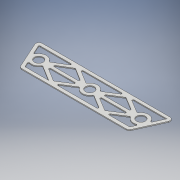
# Autodesk Inventor part: 6wdPlateInner
Saved by Autodesk Inventor 2018.3 (Build 223284000, 284)
## iProperties
Created: 2018-06-26
Part Number: 6wdPlateInner
Material: Generic
Document SubType Name: Modeling
Designer: mzhang
Density: 1 g/cm^3
Appearance: Default
Author: mzhang
Autodesk Inventor part; units mm, degrees
ref_plane "YZ Plane" through (0, 0, 0) normal (1, 0, 0) x (0, 1, 0)
ref_plane "XZ Plane" through (0, 0, 0) normal (0, 1, 0) x (-1, 0, 0)
ref_plane "XY Plane" through (0, 0, 0) normal (0, 0, 1) x (1, 0, 0)
sketch "Sketch1" plane through (0, 0, 0) normal (0, 0, 1) x (1, 0, 0)
  circle A0 centre (0, 0) radius 14.2875
  circle A1 centre (330.2, 0) radius 14.2875
  line L0 (-49.8896, 37.287) -> (-11.9465, -46.452)
  line L1 (-40.781, 51.4142) -> (51.1531, 51.4142) construction
  line L2 (-2.8379, -52.3248) -> (335.0491, -52.3248)
  line L3 (344.1679, -46.4293) -> (381.8605, 37.3096)
  line L4 (372.7417, 51.4142) -> (-40.781, 51.4142)
  circle A2 centre (165.1, 0) radius 14.2875
  arc A3 (-40.781, 51.4142) -> (-49.8896, 37.287) centre (-40.781, 41.4142) ccw
  arc A4 (-11.9465, -46.452) -> (-2.8379, -52.3248) centre (-2.8379, -42.3248) ccw
  arc A5 (335.0491, -52.3248) -> (344.1679, -46.4293) centre (335.0491, -42.3248) ccw
  arc A6 (381.8605, 37.3096) -> (372.7417, 51.4142) centre (372.7417, 41.4142) ccw
  line L5 (33.4321, 5) -> (131.8673, 5)
  line L6 (198.195, 5) -> (296.7702, 5)
  line L7 (33.2893, -5) -> (132.005, -5)
  line L8 (198.5298, -5) -> (297.105, -5)
  line L9 (330.2, 0) -> (315.9125, 0)
  arc A7 (-5.925, -23.5537) -> (20.7741, -12.5825) centre (0, 0) ccw
  arc A8 (20.7925, 12.5521) -> (-21.6765, 10.9549) centre (0, 0) ccw
  line L10 (0, 0) -> (14.2875, 0)
  arc A9 (142.9266, -9.9107) -> (187.2845, -9.886) centre (165.1, 0) ccw
  arc A10 (187.2734, 9.9107) -> (142.9218, 9.9) centre (165.1, 0) ccw
  arc A11 (354.4734, 0.8287) -> (308.0155, 9.886) centre (330.2, 0) ccw
  arc A12 (308.0266, -9.9107) -> (345.6741, -18.7199) centre (330.2, 0) ccw
  line L11 (372.7424, 41.7007) -> (354.4734, 0.8287)
  line L12 (345.6741, -18.7199) -> (335.1217, -41.2193)
  line L13 (-3.5725, -40.2425) -> (-9.3784, -27.7254)
  line L14 (-27.0783, 11.0519) -> (-38.8215, 36.5186)
  line L15 (24.9128, 11.5352) -> (64.4421, 35.4317)
  line L16 (92.8242, 41.0668) -> (142.9218, 9.9)
  line L17 (33.4321, 5) -> (83.3557, 35.1801)
  line L18 (83.3557, 35.1801) -> (131.8673, 5)
  line L19 (33.2893, -5) -> (83.3551, -35.8908)
  line L20 (83.3551, -35.8908) -> (132.005, -5)
  line L21 (24.9154, -11.5836) -> (73.9059, -41.8109)
  line L22 (92.7543, -41.7682) -> (142.9266, -9.9107)
  line L23 (187.2734, 9.9107) -> (236.8547, 41.393)
  line L24 (255.8424, 41.436) -> (308.0155, 9.886)
  line L25 (198.195, 5) -> (246.2801, 35.5322)
  line L26 (246.2801, 35.5322) -> (296.7702, 5)
  line L27 (198.5298, -5) -> (249.0199, -35.5322)
  line L28 (249.0199, -35.5322) -> (297.105, -5)
  line L29 (187.2845, -9.886) -> (239.4576, -41.436)
  line L30 (258.4453, -41.393) -> (308.0266, -9.9107)
  line L31 (-36.104, 40.7748) -> (62.8833, 40.999)
  line L32 (92.8242, 41.0668) -> (372.7424, 41.7007)
  line L33 (335.1217, -41.2193) -> (258.4453, -41.393)
  arc A13 (-27.0783, 11.0519) -> (-21.6765, 10.9549) centre (-24.354, 12.3081) ccw
  arc A14 (-36.104, 40.7748) -> (-38.8215, 36.5186) centre (-36.0972, 37.7748) ccw
  arc A15 (64.4421, 35.4317) -> (62.8833, 40.999) centre (62.8901, 37.999) ccw
  arc A16 (20.7925, 12.5521) -> (24.9128, 11.5352) centre (23.3608, 14.1025) ccw
  arc A17 (24.9154, -11.5836) -> (20.7741, -12.5825) centre (23.3401, -14.1367) ccw
  arc A18 (-5.925, -23.5537) -> (-9.3784, -27.7254) centre (-6.6569, -26.4631) ccw
  arc A19 (-3.5725, -40.2425) -> (-0.8442, -41.9802) centre (-0.851, -38.9802) ccw
  line L34 (239.4576, -41.436) -> (92.7543, -41.7682)
  line L35 (73.9059, -41.8109) -> (-0.8442, -41.9802)
  point P0 (-23.9208, 4.2044)
  point P1 (-12.6105, -20.7571)
  point P2 (22.1801, -9.8958)
  point P3 (22.1845, 9.8858)
  dimension "d0" = 28.575
  dimension "d9" = 10
  dimension "d22" = 3
  constraints: 72 end point, 38 point on circle, 23 tangent, 18 centre point, 13 parallel, 9 equal radius, 6 point on line, 2 horizontal, 2 horizontal alignment, 1 coincident, 1 equal length, 4 other
  measures "d9" radius of A3
  measures "d22" radius of A13
extrude "Extrusion1" add sketch "Sketch1" along normal blind 3.175
fillet "Fillet1" radius 3 26 edges at (33.4321, 5, 1.5875) (83.3557, 35.1801, 1.5875) (131.8673, 5, 1.5875) (33.2893, -5, 1.5875) (132.005, -5, 1.5875) (83.3551, -35.8908, 1.5875) (92.7543, -41.7682, 1.5875) (142.9266, -9.9107, 1.5875) (142.9218, 9.9, 1.5875) (92.8242, 41.0668, 1.5875) (236.8547, 41.393, 1.5875) (239.4576, -41.436, 1.5875) (187.2845, -9.886, 1.5875) (187.2734, 9.9107, 1.5875) (246.2801, 35.5322, 1.5875) (198.195, 5, 1.5875) (198.5298, -5, 1.5875) (249.0199, -35.5322, 1.5875) (296.7702, 5, 1.5875) (297.105, -5, 1.5875) (308.0155, 9.886, 1.5875) (354.4734, 0.8287, 1.5875) (345.6741, -18.7199, 1.5875) (308.0266, -9.9107, 1.5875) (255.8424, 41.436, 1.5875) (258.4453, -41.393, 1.5875)
body "Solid1"
